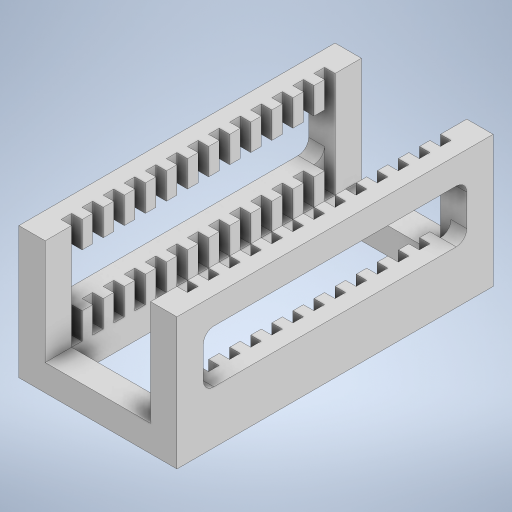
# Autodesk Inventor part: RectangularTeflonHolder
Saved by Autodesk Inventor 2023 (Build 270158000, 158)
## iProperties
Created: 2023-08-11
Part Number: RectangularTeflonHolder
Material: Generic
Document SubType Name: Modeling
Designer: Edwin
Density: 1 g/cm^3
Appearance: Default
Author: Edwin
Autodesk Inventor part; units mm, degrees
ref_plane "YZ Plane" through (0, 0, 0) normal (1, 0, 0) x (0, 1, 0)
ref_plane "XZ Plane" through (0, 0, 0) normal (0, 1, 0) x (-1, 0, 0)
ref_plane "XY Plane" through (0, 0, 0) normal (0, 0, 1) x (1, 0, 0)
sketch "Sketch1" plane through (0, 0, 0) normal (0, 1, 0) x (-1, 0, 0)
  line L0 (0, 0) -> (30, 0)
  line L1 (30, 0) -> (30, -60)
  line L2 (30, -60) -> (0, -60)
  line L3 (0, -60) -> (0, 0)
  line L4 (5, -5) -> (25, -5)
  line L5 (25, -5) -> (25, -55)
  line L6 (25, -55) -> (5, -55)
  line L7 (5, -55) -> (5, -5)
  point P0 (25, -30)
  dimension "d0" = 30
  dimension "d1" = 5
  dimension "d2" = 5
  dimension "d3" = 5
  dimension "d4" = 5
  dimension "d5" = 60
  constraints: 16 end point, 4 parallel, 2 horizontal, 2 perpendicular, 1 midpoint
  measures "d0" distance of L0.start L0.end
  measures "d1" distance between parallel lines of L3 L7
  measures "d2" distance from line of L1 point (25, -30)
  measures "d3" distance between parallel lines of L0 L4
  measures "d4" distance between parallel lines of L2 L6
  measures "d5" distance of L2.end L0.start
extrude "Extrusion1" add sketch "Sketch1" along normal blind 5
sketch "Sketch2" plane through (0, 5, 0) normal (0, 1, 0) x (1, 0, 0)
  line L0 (-30, 0) -> (0, 0) projected
  line L1 (0, 60) -> (-30, 60) projected
  line L2 (0, 0) -> (-5, 0)
  line L3 (-5, 55) -> (-5, 5) projected
  line L4 (-5, 0) -> (-5, 5)
  line L5 (-5, 5) -> (-3, 5)
  line L6 (-3, 5) -> (-3, 7)
  line L7 (-3, 7) -> (-5, 7)
  line L8 (-5, 7) -> (-5, 9)
  line L9 (-5, 9) -> (-3, 9)
  line L10 (-3, 9) -> (-3, 11)
  line L11 (-3, 11) -> (-5, 11)
  line L12 (-5, 11) -> (-5, 13)
  line L13 (-5, 13) -> (-3, 13)
  line L14 (-3, 13) -> (-3, 15)
  line L15 (-3, 15) -> (-5, 15)
  line L16 (-5, 15) -> (-5, 17)
  line L17 (-5, 17) -> (-3, 17)
  line L18 (-3, 17) -> (-3, 19)
  line L19 (-3, 19) -> (-5, 19)
  line L20 (-5, 19) -> (-5, 21)
  line L21 (-5, 21) -> (-3, 21)
  line L22 (-3, 21) -> (-3, 23)
  line L23 (-3, 23) -> (-5, 23)
  line L24 (-5, 23) -> (-5, 25)
  line L25 (-5, 25) -> (-3, 25)
  line L26 (-3, 25) -> (-3, 27)
  line L27 (-3, 27) -> (-5, 27)
  line L28 (-5, 27) -> (-5, 29)
  line L29 (-5, 29) -> (-3, 29)
  line L30 (-3, 29) -> (-3, 31)
  line L31 (-3, 31) -> (-5, 31)
  line L32 (-5, 31) -> (-5, 33)
  line L33 (-5, 33) -> (-3, 33)
  line L34 (-3, 33) -> (-3, 35)
  line L35 (-3, 35) -> (-5, 35)
  line L36 (-5, 35) -> (-5, 37)
  line L37 (-5, 37) -> (-3, 37)
  line L38 (-3, 37) -> (-3, 39)
  line L39 (-3, 39) -> (-5, 39)
  line L40 (-5, 39) -> (-5, 41)
  line L41 (-5, 41) -> (-3, 41)
  line L42 (-3, 41) -> (-3, 43)
  line L43 (-3, 43) -> (-5, 43)
  line L44 (-5, 43) -> (-5, 45)
  line L45 (-5, 45) -> (-3, 45)
  line L46 (-3, 45) -> (-3, 47)
  line L47 (-3, 47) -> (-5, 47)
  line L48 (-5, 47) -> (-5, 49)
  line L49 (-5, 49) -> (-3, 49)
  line L50 (-3, 49) -> (-3, 51)
  line L51 (-3, 51) -> (-5, 51)
  line L52 (-5, 51) -> (-5, 53)
  line L53 (-15, 0) -> (-15, 60) construction
  line L54 (0, 0) -> (0, 60) projected
  line L55 (-5, 60) -> (0, 60)
  line L56 (0, 60) -> (0, 0)
  line L57 (-5, 53) -> (-3, 53)
  line L58 (-3, 53) -> (-3, 55)
  line L59 (-3, 55) -> (-5, 55)
  line L60 (-5, 55) -> (-5, 57)
  line L61 (-5, 57) -> (-5, 60)
  line L62 (-30, 0) -> (-25, 0)
  line L63 (-25, 55) -> (-25, 5)
  line L64 (-25, 0) -> (-25, 5)
  line L65 (-25, 5) -> (-27, 5)
  line L66 (-27, 5) -> (-27, 7)
  line L67 (-27, 7) -> (-25, 7)
  line L68 (-25, 7) -> (-25, 9)
  line L69 (-25, 9) -> (-27, 9)
  line L70 (-27, 9) -> (-27, 11)
  line L71 (-27, 11) -> (-25, 11)
  line L72 (-25, 11) -> (-25, 13)
  line L73 (-25, 13) -> (-27, 13)
  line L74 (-27, 13) -> (-27, 15)
  line L75 (-27, 15) -> (-25, 15)
  line L76 (-25, 15) -> (-25, 17)
  line L77 (-25, 17) -> (-27, 17)
  line L78 (-27, 17) -> (-27, 19)
  line L79 (-27, 19) -> (-25, 19)
  line L80 (-25, 19) -> (-25, 21)
  line L81 (-25, 21) -> (-27, 21)
  line L82 (-27, 21) -> (-27, 23)
  line L83 (-27, 23) -> (-25, 23)
  line L84 (-25, 23) -> (-25, 25)
  line L85 (-25, 25) -> (-27, 25)
  line L86 (-27, 25) -> (-27, 27)
  line L87 (-27, 27) -> (-25, 27)
  line L88 (-25, 27) -> (-25, 29)
  line L89 (-25, 29) -> (-27, 29)
  line L90 (-27, 29) -> (-27, 31)
  line L91 (-27, 31) -> (-25, 31)
  line L92 (-25, 31) -> (-25, 33)
  line L93 (-25, 33) -> (-27, 33)
  line L94 (-27, 33) -> (-27, 35)
  line L95 (-27, 35) -> (-25, 35)
  line L96 (-25, 35) -> (-25, 37)
  line L97 (-25, 37) -> (-27, 37)
  line L98 (-27, 37) -> (-27, 39)
  line L99 (-27, 39) -> (-25, 39)
  line L100 (-25, 39) -> (-25, 41)
  line L101 (-25, 41) -> (-27, 41)
  line L102 (-27, 41) -> (-27, 43)
  line L103 (-27, 43) -> (-25, 43)
  line L104 (-25, 43) -> (-25, 45)
  line L105 (-25, 45) -> (-27, 45)
  line L106 (-27, 45) -> (-27, 47)
  line L107 (-27, 47) -> (-25, 47)
  line L108 (-25, 47) -> (-25, 49)
  line L109 (-25, 49) -> (-27, 49)
  line L110 (-27, 49) -> (-27, 51)
  line L111 (-27, 51) -> (-25, 51)
  line L112 (-25, 51) -> (-25, 53)
  line L113 (-30, 0) -> (-30, 60)
  line L114 (-25, 60) -> (-30, 60)
  line L115 (-30, 60) -> (-30, 0)
  line L116 (-25, 53) -> (-27, 53)
  line L117 (-27, 53) -> (-27, 55)
  line L118 (-27, 55) -> (-25, 55)
  line L119 (-25, 55) -> (-25, 57)
  line L120 (-25, 57) -> (-25, 60)
  point P0 (-5, 25)
  point P1 (-5, 29)
  point P2 (-5, 33)
  point P3 (-5, 37)
  point P4 (-5, 41)
  point P5 (-5, 45)
  point P6 (-5, 49)
  point P7 (-5, 7)
  point P8 (-5, 51)
  point P9 (-5, 49)
  point P10 (-5, 47)
  point P11 (-5, 45)
  point P12 (-5, 43)
  point P13 (-5, 41)
  point P14 (-5, 39)
  point P15 (-5, 35)
  point P16 (-5, 33)
  point P17 (-5, 31)
  point P18 (-5, 29)
  point P19 (-5, 27)
  point P20 (-5, 21)
  point P21 (-5, 19)
  point P22 (-5, 15)
  point P23 (-5, 13)
  point P24 (-5, 11)
  point P25 (-5, 9)
  point P26 (-5, 53)
  point P27 (-25, 29)
  point P28 (-25, 33)
  point P29 (-25, 37)
  dimension "d8" = 5
  dimension "d9" = 2
  dimension "d10" = 2
  dimension "d11" = 2
  dimension "d14" = 4
  constraints: 234 end point, 81 symmetric about line, 72 vertical alignment, 24 collinear, 24 parallel, 5 perpendicular, 5 point on line, 3 vertical, 2 midpoint, 1 horizontal, 1 other
  measures "d8" distance of L2.end L4.end
  measures "d9" distance of L4.end L5.end
  measures "d10" distance of L5.end L6.end
  measures "d11" distance of L7.end L8.end
  measures "d14" distance of point (-5, 5) point (-5, 9)
extrude "Extrusion2" add sketch "Sketch2" along normal blind 20 contours L113 L1 L120 L119 L118 L117 L116 L63 L111 L110 L109 L107 L106 L105 L103 L102 L101 L99 L98 L97 L95 L94 L93 L91 L90 L89 L87 L86 L85 L83 L82 L81 L79 L78 L77 L75 L74 L73 L71 L70 L69 L67 L66 L65 L64 L0 | L4 L5 L6 L7 L3 L9 L10 L11 L13 L14 L15 L17 L18 L19 L21 L22 L23 L25 L26 L27 L29 L30 L31 L33 L34 L35 L37 L38 L39 L41 L42 L43 L45 L46 L47 L49 L50 L51 L57 L58 L59 L60 L61 L1 L54 L0
sketch "Sketch3" plane through (0, 0, 0) normal (1, 0, 0) x (0, 0, -1)
  line L0 (7, 10) -> (53, 10)
  line L1 (55, 12) -> (55, 18)
  line L2 (53, 20) -> (7, 20)
  line L3 (5, 18) -> (5, 12)
  line L4 (0, 0) -> (60, 0) projected
  line L5 (0, 25) -> (60, 25) projected
  line L6 (0, 0) -> (0, 25) projected
  line L7 (60, 0) -> (60, 25) projected
  arc A0 (7, 20) -> (5, 18) centre (7, 18) ccw
  arc A1 (5, 12) -> (7, 10) centre (7, 12) ccw
  arc A2 (53, 10) -> (55, 12) centre (53, 12) ccw
  arc A3 (55, 18) -> (53, 20) centre (53, 18) ccw
  point P0 (5, 5)
  point P1 (5, 10)
  point P2 (55, 20)
  point P3 (55, 10)
  point P4 (5, 20)
  dimension "d21" = 10
  dimension "d22" = 5
  dimension "d23" = 5
  dimension "d24" = 5
  dimension "d27" = 2
  constraints: 8 end point, 8 point on circle, 8 point on line, 8 tangent, 4 centre point, 3 equal radius, 2 parallel, 1 horizontal, 1 perpendicular
  measures "d21" distance between parallel lines of L4 L0
  measures "d22" distance between parallel lines of L5 L2
  measures "d23" distance between parallel lines of L6 L3
  measures "d24" distance between parallel lines of L7 L1
  measures "d27" radius of A0
extrude "Extrusion3" cut sketch "Sketch3" against normal blind 40 contours A1 L3 A0 L2 A3 L1 A2 L0
body "Solid1"
